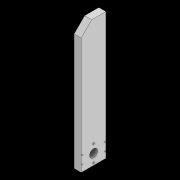
# Autodesk Inventor part: launcherV2
Saved by Autodesk Inventor 2022 (Build 260153000, 153)
## iProperties
Created: 2021-10-08
Part Number: launcherV2
Material: Generic
Document SubType Name: Modeling
Designer: timmy
Density: 1 g/cm^3
Appearance: Default
Author: timmy
Autodesk Inventor part; units mm, degrees
ref_plane "YZ Plane" through (0, 0, 0) normal (1, 0, 0) x (0, 1, 0)
ref_plane "XZ Plane" through (0, 0, 0) normal (0, 1, 0) x (-1, 0, 0)
ref_plane "XY Plane" through (0, 0, 0) normal (0, 0, 1) x (1, 0, 0)
sketch "Sketch1" plane through (0, 0, 0) normal (1, 0, 0) x (0, 1, 0)
  line L0 (0, 0) -> (76.2, 0)
  line L1 (76.2, 0) -> (76.2, -88.9)
  line L2 (76.2, -88.9) -> (0, -88.9)
  line L3 (0, -88.9) -> (0, 0)
  dimension "d0" = 76.2
  dimension "d1" = 88.9
  constraints: 8 end point, 2 parallel, 1 horizontal, 1 perpendicular
  measures "d0" distance of L1.end L2.end
  measures "d1" distance of L0.end L1.end
extrude "Extrusion1" add sketch "Sketch1" along normal blind 25.4
sketch "Sketch2" plane through (25.4, 0, 0) normal (1, 0, 0) x (0, 0, -1)
  line L0 (88.9, 76.2) -> (0, 76.2) projected
  line L1 (44.45, 76.2) -> (44.45, 0)
  line L2 (0, 0) -> (88.9, 0) projected
  circle A0 centre (44.45, 38.1) radius 14.2875
  line L3 (44.45, 38.1) -> (3.7084, 38.1)
  circle A1 centre (3.7084, 52.832) radius 2.0193
  circle A2 centre (3.7084, 23.368) radius 2.0193
  circle A3 centre (85.1916, 52.832) radius 2.0193
  circle A4 centre (85.1916, 23.368) radius 2.0193
  line L4 (44.45, 38.1) -> (44.45, 68.0212)
  circle A5 centre (44.45, 68.0212) radius 3.302
  circle A6 centre (44.45, 8.1788) radius 3.302
  point P0 (85.1916, 38.1)
  dimension "d4" = 28.575
  dimension "d5" = 40.7416
  dimension "d8" = 29.9212
  dimension "d9" = 6.604
  constraints: 7 centre point, 6 end point, 5 symmetric about line, 3 midpoint, 1 coincident, 1 horizontal, 1 point on line, 4 other
  measures "d4" diameter of A0
  measures "d5" distance of L3.start L3.end
  measures "d8" distance of L3.start L4.end
  measures "d9" diameter of A5
extrude "Extrusion2" cut sketch "Sketch2" against normal up to surface (25.4 mm away)
sketch "Sketch3" plane through (0, 76.2, 0) normal (0, 1, 0) x (1, 0, 0)
  line L0 (0, 88.9) -> (0, 0) projected
  line L1 (0, 0) -> (25.4, 0) projected
  line L2 (25.4, 88.9) -> (25.4, 0) projected
  line L3 (0, 88.9) -> (25.4, 88.9) projected
extrude "Extrusion3" add sketch "Sketch3" along normal blind 381
chamfer "Chamfer1" distance 38.1 angle 45 1 edges at (12.7, 457.2, 0)
body "Solid1"
